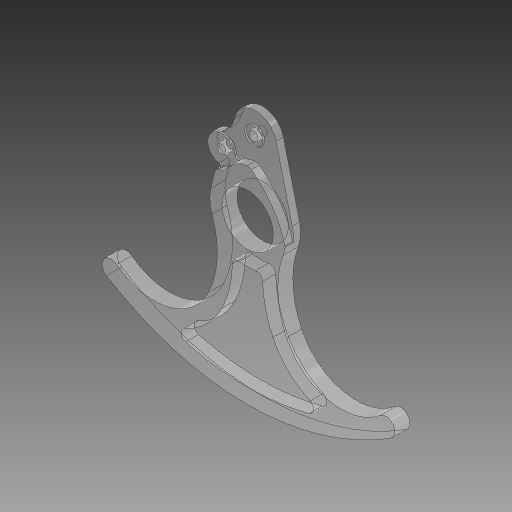
# Autodesk Inventor part: ヘッケン2
Saved by Autodesk Inventor 2020 (Build 240168000, 168)
## iProperties
Created: 2019-09-03
Part Number: ヘッケン2
Material: ポリカーボネート、クリア
Document SubType Name: Modeling
Designer: 雪村
Density: 1.2 g/cm^3
Appearance: ポリカーボネート - クリア
Mass: 9.36853 g
Surface Area: 71.3184 cm^2
Volume: 7.80711 cm^3
Description: ポリカ 5t
Author: 雪村
Autodesk Inventor part; units mm, degrees
ref_plane "YZ Plane" through (0, 0, 0) normal (1, 0, 0) x (0, 1, 0)
ref_plane "XZ Plane" through (0, 0, 0) normal (0, 1, 0) x (-1, 0, 0)
ref_plane "XY Plane" through (0, 0, 0) normal (0, 0, 1) x (1, 0, 0)
sketch "スケッチ1" plane through (0, 0, 0) normal (0, 0, 1) x (1, 0, 0)
  spline S0 degree 4 poles (47.3109, -61.9649) (47.0065, -62.1545) (46.5798, -62.4175) (46.0301, -62.7516) (45.3565, -63.1534) (44.8664, -63.4421) (44.3758, -63.7275) (43.8846, -64.0096) (43.3928, -64.2883) (42.9004, -64.5638) (42.4073, -64.8361) (41.9135, -65.1051) (41.419, -65.3708) (40.9238, -65.6334) (40.4279, -65.8927) (39.9312, -66.1487) (39.4337, -66.4016) (38.9355, -66.6513) (38.4364, -66.8977) (37.9366, -67.141) (37.4359, -67.381) (36.9344, -67.6179) (36.432, -67.8515) (35.9288, -68.082) (35.4247, -68.3093) (34.9198, -68.5333) (34.414, -68.7542) (33.9073, -68.9719) (33.3998, -69.1863) (32.8914, -69.3976) (32.3821, -69.6056) (31.8719, -69.8105) (31.3609, -70.0121) (30.849, -70.2105) (30.3362, -70.4056) (29.8225, -70.5976) (29.308, -70.7863) (28.7926, -70.9717) (28.2764, -71.1539) (27.7593, -71.3329) (27.2413, -71.5086) (26.7225, -71.681) (26.2029, -71.8502) (25.6825, -72.016) (25.1612, -72.1786) (24.6392, -72.3379) (24.1163, -72.4939) (23.5927, -72.6466) (23.0683, -72.796) (22.5431, -72.942) (22.0172, -73.0848) (21.4905, -73.2242) (20.9632, -73.3602) (20.4351, -73.4929) (19.9062, -73.6223) (19.3768, -73.7483) (18.8466, -73.8709) (18.3158, -73.9902) (17.7843, -74.1061) (17.2522, -74.2186) (16.7195, -74.3277) (16.1862, -74.4334) (15.6524, -74.5357) (15.1179, -74.6346) (14.5829, -74.73) (14.0474, -74.8221) (13.5114, -74.9107) (12.9749, -74.9959) (12.4379, -75.0777) (11.9005, -75.156) (11.3626, -75.2309) (10.8243, -75.3023) (10.2856, -75.3703) (9.7465, -75.4348) (9.207, -75.4958) (8.6672, -75.5534) (8.1271, -75.6075) (7.5867, -75.6581) (7.046, -75.7053) (6.505, -75.749) (5.9638, -75.7892) (5.4223, -75.8259) (4.8807, -75.8591) (4.3389, -75.8888) (3.7969, -75.915) (3.2547, -75.9378) (2.7124, -75.957) (2.1701, -75.9728) (1.6276, -75.985) (1.0851, -75.9937) (0.5426, -75.999) (0, -76.0007) (-0.5426, -75.999) (-1.0851, -75.9937) (-1.6276, -75.985) (-2.1701, -75.9728) (-2.7125, -75.957) (-3.2547, -75.9378) (-3.7969, -75.915) (-4.3389, -75.8888) (-4.8807, -75.8591) (-5.4224, -75.8259) (-5.9638, -75.7892) (-6.505, -75.749) (-7.046, -75.7053) (-7.5868, -75.6581) (-8.1272, -75.6075) (-8.6674, -75.5534) (-9.2072, -75.4958) (-9.7467, -75.4348) (-10.2859, -75.3703) (-10.8247, -75.3023) (-11.363, -75.2308) (-11.901, -75.156) (-12.4386, -75.0776) (-12.9757, -74.9959) (-13.5124, -74.9106) (-14.0486, -74.822) (-14.5843, -74.7299) (-15.1195, -74.6344) (-15.6541, -74.5355) (-16.1883, -74.4331) (-16.7219, -74.3274) (-17.2549, -74.2182) (-17.7874, -74.1057) (-18.3193, -73.9897) (-18.8505, -73.8704) (-19.3812, -73.7477) (-19.9113, -73.6216) (-20.4407, -73.4921) (-20.9695, -73.3593) (-21.4976, -73.2231) (-22.0251, -73.0835) (-22.5519, -72.9406) (-23.078, -72.7943) (-23.6035, -72.6447) (-24.1283, -72.4918) (-24.6524, -72.3355) (-25.1758, -72.1759) (-25.6985, -72.0129) (-26.2205, -71.8466) (-26.7418, -71.6771) (-27.2625, -71.5041) (-27.7825, -71.3279) (-28.3017, -71.1484) (-28.8203, -70.9655) (-29.3383, -70.7793) (-29.8555, -70.5898) (-30.3721, -70.397) (-30.8881, -70.2009) (-31.4034, -70.0014) (-31.9181, -69.7986) (-32.4322, -69.5925) (-32.9457, -69.3831) (-33.4587, -69.1703) (-33.9711, -68.9541) (-34.483, -68.7346) (-34.9944, -68.5118) (-35.5054, -68.2855) (-36.0159, -68.0558) (-36.526, -67.8228) (-37.0357, -67.5863) (-37.5452, -67.3463) (-38.0543, -67.1029) (-38.5633, -66.8559) (-39.072, -66.6054) (-39.5807, -66.3514) (-40.0892, -66.0938) (-40.5978, -65.8326) (-41.1064, -65.5676) (-41.6152, -65.299) (-42.1242, -65.0266) (-42.6335, -64.7504) (-43.1431, -64.4703) (-43.6533, -64.1863) (-44.164, -63.8983) (-44.6755, -63.6062) (-45.3809, -63.1982) (-45.9582, -62.8581) (-46.4075, -62.5897) (-46.7287, -62.3958) knots 0 0 0 0 0 0.014153 0.019804 0.025448 0.031087 0.03672 0.042347 0.047969 0.053586 0.059197 0.064804 0.070407 0.076005 0.081599 0.087189 0.092776 0.098358 0.103937 0.109513 0.115086 0.120655 0.126222 0.131786 0.137347 0.142906 0.148462 0.154016 0.159567 0.165117 0.170664 0.17621 0.181753 0.187295 0.192835 0.198374 0.203911 0.209447 0.214981 0.220514 0.226045 0.231576 0.237105 0.242633 0.24816 0.253686 0.259211 0.264735 0.270259 0.275781 0.281303 0.286824 0.292344 0.297864 0.303383 0.308902 0.31442 0.319937 0.325454 0.33097 0.336486 0.342002 0.347517 0.353031 0.358546 0.36406 0.369573 0.375087 0.3806 0.386112 0.391625 0.397137 0.402649 0.408161 0.413673 0.419184 0.424696 0.430207 0.435718 0.441229 0.446739 0.45225 0.457761 0.463271 0.468782 0.474292 0.479802 0.485312 0.490823 0.496333 0.501843 0.507353 0.512863 0.518373 0.523883 0.529394 0.534904 0.540414 0.545925 0.551435 0.556946 0.562456 0.567967 0.573478 0.578989 0.584501 0.590012 0.595524 0.601036 0.606548 0.61206 0.617573 0.623086 0.628599 0.634113 0.639627 0.645141 0.650656 0.656172 0.661687 0.667204 0.672721 0.678238 0.683757 0.689275 0.694795 0.700315 0.705837 0.711359 0.716882 0.722406 0.727931 0.733457 0.738984 0.744513 0.750043 0.755574 0.761107 0.766641 0.772178 0.777715 0.783255 0.788797 0.794341 0.799887 0.805435 0.810986 0.816539 0.822096 0.827655 0.833217 0.838783 0.844352 0.849924 0.855501 0.861082 0.866667 0.872256 0.877851 0.88345 0.889055 0.894666 0.900282 0.905905 0.911535 0.917171 0.922816 0.928468 0.934129 0.939798 0.945477 0.951166 0.956865 0.962575 0.968297 0.974032 0.979779 0.985541 1 1 1 1 1
  circle A0 centre (0, 0) radius 1.5
  circle A1 centre (0, -23) radius 8.525
  circle A2 centre (0, 0) radius 7.025
  circle A3 centre (0, -23) radius 12.525
  line L0 (-6.8212, 1.6799) -> (-12.1616, -20.0049)
  line L1 (6.8212, 1.6799) -> (12.1616, -20.0049)
  arc A4 (-43.3371, -57.4602) -> (-46.7287, -62.3958) centre (-45.1853, -59.8233) ccw
  arc A5 (47.3109, -61.9649) -> (43.8031, -57.1163) centre (45.732, -59.414) ccw
  line L2 (-46.7287, -62.3958) -> (-46.2133, -62.705) construction
  line L3 (46.8227, -62.2671) -> (47.3109, -61.9649) construction
  arc A6 (-43.3371, -57.4602) -> (-12.9977, -50.3865) centre (-31.0158, -41.7063) ccw
  arc A7 (-12.9977, -50.3865) -> (-11.7886, -27.2313) centre (-40.0249, -37.3662) ccw
  arc A8 (11.7739, -27.272) -> (12.8817, -50.3865) centre (39.975, -37.5042) ccw
  arc A9 (12.8817, -50.3865) -> (43.8031, -57.1163) centre (30.9439, -41.7983) ccw
  line L4 (-46.7287, -62.3958) -> (0, -23) construction
  line L5 (47.3109, -61.9649) -> (0, -23) construction
  line L6 (0, -23) -> (0, -76) construction
  point P0 (46.3342, -62.5658)
  point P1 (45.8451, -62.8612)
  point P2 (45.3556, -63.1532)
  point P3 (44.8656, -63.4419)
  point P4 (44.375, -63.7272)
  point P5 (43.8838, -64.0093)
  point P6 (43.392, -64.288)
  point P7 (42.8996, -64.5635)
  point P8 (42.4065, -64.8358)
  point P9 (41.9128, -65.1047)
  point P10 (41.4183, -65.3705)
  point P11 (40.9231, -65.633)
  point P12 (40.4272, -65.8923)
  point P13 (39.9305, -66.1483)
  point P14 (39.4331, -66.4012)
  point P15 (38.9348, -66.6508)
  point P16 (38.4358, -66.8973)
  point P17 (37.936, -67.1405)
  point P18 (37.4353, -67.3805)
  point P19 (36.9338, -67.6174)
  point P20 (36.4314, -67.851)
  point P21 (35.9282, -68.0815)
  point P22 (35.4242, -68.3087)
  point P23 (34.9193, -68.5328)
  point P24 (34.4135, -68.7537)
  point P25 (33.9068, -68.9713)
  point P26 (33.3993, -69.1858)
  point P27 (32.8909, -69.397)
  point P28 (32.3816, -69.6051)
  point P29 (31.8715, -69.8099)
  point P30 (31.3605, -70.0115)
  point P31 (30.8485, -70.2099)
  point P32 (30.3358, -70.4051)
  point P33 (29.8221, -70.597)
  point P34 (29.3076, -70.7857)
  point P35 (28.7922, -70.9711)
  point P36 (28.276, -71.1533)
  point P37 (27.7589, -71.3323)
  point P38 (27.241, -71.508)
  point P39 (26.7222, -71.6804)
  point P40 (26.2026, -71.8495)
  point P41 (25.6822, -72.0154)
  point P42 (25.1609, -72.178)
  point P43 (24.6389, -72.3373)
  point P44 (24.1161, -72.4933)
  point P45 (23.5924, -72.6459)
  point P46 (23.068, -72.7953)
  point P47 (22.5429, -72.9414)
  point P48 (22.0169, -73.0841)
  point P49 (21.4903, -73.2235)
  point P50 (20.9629, -73.3596)
  point P51 (20.4348, -73.4923)
  point P52 (19.906, -73.6216)
  point P53 (19.3765, -73.7476)
  point P54 (18.8464, -73.8702)
  point P55 (18.3156, -73.9895)
  point P56 (17.7841, -74.1054)
  point P57 (17.252, -74.2179)
  point P58 (16.7193, -74.327)
  point P59 (16.1861, -74.4327)
  point P60 (15.6522, -74.535)
  point P61 (15.1178, -74.6339)
  point P62 (14.5828, -74.7293)
  point P63 (14.0473, -74.8214)
  point P64 (13.5113, -74.91)
  point P65 (12.9748, -74.9952)
  point P66 (12.4378, -75.077)
  point P67 (11.9003, -75.1553)
  point P68 (11.3625, -75.2302)
  point P69 (10.8242, -75.3016)
  point P70 (10.2855, -75.3696)
  point P71 (9.7464, -75.4341)
  point P72 (9.2069, -75.4951)
  point P73 (8.6671, -75.5527)
  point P74 (8.127, -75.6068)
  point P75 (7.5866, -75.6574)
  point P76 (7.0459, -75.7046)
  point P77 (6.5049, -75.7482)
  point P78 (5.9637, -75.7884)
  point P79 (5.4223, -75.8251)
  point P80 (4.8806, -75.8583)
  point P81 (4.3388, -75.8881)
  point P82 (3.7968, -75.9143)
  point P83 (3.2547, -75.937)
  point P84 (2.7124, -75.9563)
  point P85 (2.1701, -75.972)
  point P86 (1.6276, -75.9843)
  point P87 (1.0851, -75.993)
  point P88 (0.5426, -75.9983)
  point P89 (-0.5426, -75.9983)
  point P90 (-1.0851, -75.993)
  point P91 (-1.6276, -75.9843)
  point P92 (-2.1701, -75.972)
  point P93 (-2.7124, -75.9563)
  point P94 (-3.2547, -75.937)
  point P95 (-3.7968, -75.9143)
  point P96 (-4.3388, -75.8881)
  point P97 (-4.8806, -75.8583)
  point P98 (-5.4223, -75.8251)
  point P99 (-5.9637, -75.7884)
  point P100 (-6.505, -75.7482)
  point P101 (-7.046, -75.7046)
  point P102 (-7.5867, -75.6574)
  point P103 (-8.1271, -75.6068)
  point P104 (-8.6673, -75.5527)
  point P105 (-9.2071, -75.4951)
  point P106 (-9.7466, -75.434)
  point P107 (-10.2858, -75.3695)
  point P108 (-10.8245, -75.3016)
  point P109 (-11.3629, -75.2301)
  point P110 (-11.9009, -75.1553)
  point P111 (-12.4384, -75.0769)
  point P112 (-12.9755, -74.9951)
  point P113 (-13.5122, -74.9099)
  point P114 (-14.0484, -74.8213)
  point P115 (-14.5841, -74.7292)
  point P116 (-15.1193, -74.6337)
  point P117 (-15.6539, -74.5348)
  point P118 (-16.1881, -74.4324)
  point P119 (-16.7217, -74.3267)
  point P120 (-17.2547, -74.2175)
  point P121 (-17.7872, -74.105)
  point P122 (-18.319, -73.9891)
  point P123 (-18.8503, -73.8697)
  point P124 (-19.381, -73.747)
  point P125 (-19.911, -73.6209)
  point P126 (-20.4404, -73.4914)
  point P127 (-20.9692, -73.3586)
  point P128 (-21.4973, -73.2224)
  point P129 (-22.0248, -73.0828)
  point P130 (-22.5516, -72.9399)
  point P131 (-23.0777, -72.7937)
  point P132 (-23.6031, -72.6441)
  point P133 (-24.1279, -72.4911)
  point P134 (-24.652, -72.3348)
  point P135 (-25.1754, -72.1752)
  point P136 (-25.6981, -72.0123)
  point P137 (-26.2201, -71.846)
  point P138 (-26.7414, -71.6764)
  point P139 (-27.2621, -71.5035)
  point P140 (-27.782, -71.3273)
  point P141 (-28.3013, -71.1478)
  point P142 (-28.8199, -70.9649)
  point P143 (-29.3378, -70.7788)
  point P144 (-29.855, -70.5893)
  point P145 (-30.3716, -70.3965)
  point P146 (-30.8875, -70.2003)
  point P147 (-31.4028, -70.0009)
  point P148 (-31.9175, -69.7981)
  point P149 (-32.4316, -69.592)
  point P150 (-32.9451, -69.3826)
  point P151 (-33.458, -69.1698)
  point P152 (-33.9704, -68.9537)
  point P153 (-34.4823, -68.7342)
  point P154 (-34.9937, -68.5113)
  point P155 (-35.5046, -68.2851)
  point P156 (-36.0151, -68.0554)
  point P157 (-36.5252, -67.8224)
  point P158 (-37.0349, -67.5859)
  point P159 (-37.5443, -67.346)
  point P160 (-38.0534, -67.1025)
  point P161 (-38.5623, -66.8556)
  point P162 (-39.071, -66.6052)
  point P163 (-39.5796, -66.3512)
  point P164 (-40.0881, -66.0936)
  point P165 (-40.5967, -65.8324)
  point P166 (-41.1053, -65.5675)
  point P167 (-41.614, -65.2989)
  point P168 (-42.1229, -65.0265)
  point P169 (-42.6321, -64.7504)
  point P170 (-43.1417, -64.4703)
  point P171 (-43.6518, -64.1864)
  point P172 (-44.1625, -63.8984)
  point P173 (-44.6739, -63.6064)
  point P174 (-45.186, -63.3102)
  point P175 (-45.6991, -63.0098)
  dimension "d0" = 3
  dimension "d1" = 14.05
  dimension "d2" = 23
  dimension "d3" = 17.05
  dimension "d4" = 4
  dimension "d5" = 3
  dimension "d6" = 3
  dimension "d7" = 20
  dimension "d9" = 20
  dimension "d10" = 30
  dimension "d11" = 30
  dimension "d12" = 20
  dimension "d64" = 61.291
  dimension "d65" = 61.1195
  constraints: 18 point on circle, 14 end point, 12 tangent, 10 centre point, 3 coincident, 1 horizontal alignment, 1 point on line, 1 vertical alignment, 364 other
  measures "d0" diameter of A0
  measures "d1" diameter of A2
  measures "d2" distance of A1.centre point (0, 0)
  measures "d3" diameter of A1
  measures "d4" radial gap between concentric circles of A1 A3
  measures "d5" radius of A4
  measures "d6" radius of A5
  measures "d7" radius of A6
  measures "d9" radius of A9
  measures "d10" radius of A8
  measures "d11" radius of A7
  measures "d64" distance of L3.end L4.end
  measures "d65" distance of L2.start L4.end
extrude "押し出し1" add sketch "スケッチ1" along normal blind 5
sketch "スケッチ2" plane through (0, 0, 5) normal (0, 0, 1) x (1, 0, 0)
  line L0 (0, 0) -> (-10.6688, -9.0652)
  circle A0 centre (-10.6688, -9.0652) radius 1.5
  circle A1 centre (0, 0) radius 1.5
  circle A2 centre (-10.6688, -9.0652) radius 4.025
  circle A3 centre (0, 0) radius 7.025
  arc A4 (0.3692, -7.0153) -> (-7.3502, -11.3428) centre (0.8948, -17.0015) ccw
  arc A5 (-12.3807, -5.4224) -> (-6.8636, 1.497) centre (-16.6339, 3.628) ccw
  circle A6 centre (0, -23) radius 8.525
  arc A7 (0.3955, -7.5146) -> (-6.9379, -11.6257) centre (0.8948, -17.0015) ccw
  circle A8 centre (0, 0) radius 7.525
  circle A9 centre (-10.6688, -9.0652) radius 4.525
  circle A10 centre (0, -23) radius 8.525 projected
  circle A11 centre (0, 0) radius 1.5 projected
  circle A12 centre (0, 0) radius 3
  arc A13 (6.8212, 1.6799) -> (-6.8212, 1.6799) centre (0, 0) ccw projected
  point P0 (-6.2404, -9.995)
  point P1 (-6.9379, -11.6257)
  point P2 (0.3955, -7.5146)
  point P3 (-7.5105, -0.4663)
  point P4 (-10.8715, -4.5447)
  point P5 (-5.7345, -4.8725)
  point P6 (-7.5105, -0.4663)
  point P7 (-7.6015, -6.4589)
  point P8 (-5.3534, -4.5488)
  point P9 (-10.8715, -4.5447)
  point P10 (-6.2404, -9.995)
  dimension "d15" = 14
  dimension "d16" = 3
  dimension "d17" = 8.05
  dimension "d18" = 14.05
  dimension "d19" = 10
  dimension "d20" = 10
  dimension "d21" = 5
  dimension "d23" = 0.5
  dimension "d24" = 0.5
  dimension "d25" = 0.5
  dimension "d26" = 6
  constraints: 10 point on circle, 9 centre point, 6 tangent, 5 coincident, 2 concentric, 2 end point, 6 other
  measures "d15" distance of L0.start L0.end
  measures "d16" diameter of A0
  measures "d17" diameter of A2
  measures "d18" diameter of A3
  measures "d19" radius of A5
  measures "d20" radius of A4
  measures "d23" radial gap between concentric circles of A4 A7
  measures "d26" diameter of A12
extrude "押し出し2" cut sketch "スケッチ2" against normal through all contours A0
extrude "押し出し3" add sketch "スケッチ2" against normal blind 5 contours L0 A8 A5 A3 | L0 A9 A5 A8 | L0 A2 A5 A9 | A2 | A5 A2 A4 A9
extrude "押し出し4" cut sketch "スケッチ2" against normal blind 2.6 contours A3 A4 A8 L0 | L0 A8 A5 A3 | A3 | A8 A4 A9 L0 | L0 A9 A5 A8
extrude "押し出し5" cut sketch "スケッチ2" against normal blind 2.6 contours A5 A8 A4 A3 | A8 A7 A9 A4
extrude "押し出し6" cut sketch "スケッチ2" against normal blind 2 contours A9 A4 A2 L0 | L0 A2 A5 A9 | A2 | A5 A2 A4 A9 | A0 | A12
sketch "スケッチ3" plane through (0, 0, 5) normal (0, 0, 1) x (1, 0, 0)
  circle A0 centre (0, 0) radius 1.5
  circle A1 centre (0, -23) radius 8.525
  arc A2 (13.5102, -34.0119) -> (26.3695, -30.4286) centre (20.528, -34.3308) ccw
  line L0 (26.3695, -30.4286) -> (7.5291, -2.2246)
  arc A3 (9.0465, 2.5403) -> (7.5291, -2.2246) centre (10.1892, -0.4476) ccw
  arc A4 (9.0465, 2.5403) -> (7.7583, 7.344) centre (8.1536, 4.8754) ccw
  line L1 (7.7583, 7.344) -> (-0.9526, 5.9492)
  arc A5 (-0.9526, 5.9492) -> (-2.8348, -5.3165) centre (0, 0) ccw
  arc A6 (13.5102, -34.0119) -> (-2.8348, -5.3165) centre (-17.3869, -32.6082) ccw
  circle A7 centre (0, 0) radius 4.025
  circle A8 centre (20.528, -34.3308) radius 4.025
  line L2 (8.1536, 4.8754) -> (0, 0)
  line L3 (0, 0) -> (20.528, -34.3308)
  line L4 (0, 0) -> (0, -23)
  line L5 (0, -23) -> (-14.8833, -14.7849)
  line L6 (-14.8833, -14.7849) -> (20.528, -34.3308)
  arc A9 (-1.0316, 6.4429) -> (-3.07, -5.7577) centre (0, 0) ccw
  line L7 (-1.0316, 6.4429) -> (7.6793, 7.8377)
  arc A10 (9.2251, 2.0733) -> (7.6793, 7.8377) centre (8.1536, 4.8754) ccw
  arc A11 (9.2251, 2.0733) -> (7.9449, -1.9469) centre (10.1892, -0.4476) ccw
  line L8 (7.9449, -1.9469) -> (26.7853, -30.1508)
  arc A12 (13.0108, -33.9892) -> (26.7853, -30.1508) centre (20.528, -34.3308) ccw
  arc A13 (13.0108, -33.9892) -> (-3.07, -5.7577) centre (-17.3869, -32.6082) ccw
  arc A14 (0.3955, -7.5146) -> (-6.9379, -11.6257) centre (0.8948, -17.0015) ccw projected
  arc A15 (0.3955, -7.5146) -> (7.4662, -0.9391) centre (0, 0) ccw projected
  point P0 (0, -7.6358)
  point P1 (12.9421, -30.1436)
  point P2 (13.4655, -30.4325)
  point P3 (0, -7.0289)
  point P4 (0, -7.6358)
  point P5 (0, -7.0289)
  point P6 (13.4655, -30.4325)
  point P7 (12.9421, -30.1436)
  point P8 (-0.1161, -7.5554)
  point P9 (0.6672, -7.4954)
  dimension "d37" = 8.05
  dimension "d38" = 30.929
  dimension "d39" = 8.05
  dimension "d40" = 3
  dimension "d41" = 2.5
  dimension "d42" = 3.199
  dimension "d43" = 40
  dimension "d44" = 9.5
  dimension "d45" = 90
  dimension "d46" = 33.9179
  dimension "d47" = 17
  dimension "d48" = 40.4475
  dimension "d49" = 0.5
  dimension "d50" = 2
  constraints: 20 point on circle, 18 end point, 14 centre point, 7 tangent, 2 concentric, 1 coincident, 1 collinear, 1 vertical, 8 other
  measures "d37" diameter of A7
  measures "d38" radius of A6
  measures "d39" diameter of A8
  measures "d40" radial gap between concentric circles of A2 A8
  measures "d41" radius of A4
  measures "d42" radius of A3
  measures "d43" distance of A2.centre L2.end
  measures "d44" distance of A5.centre L2.start
  measures "d45" angle of L3 L2
  measures "d46" distance of L0.start L0.end
  measures "d47" distance of L4.end L5.end
  measures "d48" distance of L5.end L3.end
  measures "d49" radial gap between concentric circles of A6 A13
  measures "d50" radial gap between concentric circles of A5 A7
extrude "押し出し7" cut sketch "スケッチ3" against normal blind 2.6 contours A7 L4 A6 A5 L1 A4 A3 A15 L3 | L3 A15 A6 L4 A7 | A15 A3 L0 A2 A6 L6 A8 L3 | L3 A8 L6 A6 A15 | L4 A14 A13 A9 L7 A10 A11 L8 A12 L6 A6 A2 L0 A3 A4 L1 A5 | A6 A15 A14 L4
sketch "スケッチ4" plane through (0, 0, 5) normal (0, 0, 1) x (1, 0, 0)
  arc A0 (-43.3371, -57.4602) -> (-12.9977, -50.3865) centre (-31.0158, -41.7063) ccw projected
  arc A1 (-43.3371, -57.4602) -> (-46.7287, -62.3958) centre (-45.1853, -59.8233) ccw projected
  spline S0 degree 5 poles (-46.7287, -62.3958) (-42.286, -65.0772) (-37.8291, -67.4223) (-33.2662, -69.4678) (-28.606, -71.1867) (-19.1173, -73.9516) (-14.2885, -74.9975) (-9.3966, -75.6914) (-4.4706, -76.0253) (5.3761, -75.9723) (10.2982, -75.5854) (15.183, -74.8391) (20.0004, -73.7422) (29.452, -70.8796) (34.0867, -69.1138) (38.6089, -67.0279) (43.0091, -64.6436) (47.3109, -61.9649) knots 0 0 0 0 0 0 0.25 0.25 0.25 0.25 0.5 0.5 0.5 0.5 0.75 0.75 0.75 0.75 1 1 1 1 1 1
  arc A2 (-12.9977, -50.3865) -> (-11.7886, -27.2313) centre (-40.0249, -37.3662) ccw projected
  arc A3 (11.7739, -27.272) -> (12.8817, -50.3865) centre (39.975, -37.5042) ccw projected
  arc A4 (12.8817, -50.3865) -> (43.8031, -57.1163) centre (30.9439, -41.7983) ccw projected
  arc A5 (47.3109, -61.9649) -> (43.8031, -57.1163) centre (45.732, -59.414) ccw projected
  circle A6 centre (0, -23) radius 8.525 projected
  circle A7 centre (0, -23) radius 13.525
  arc A8 (-8.4931, -52.5566) -> (-7.0826, -25.5422) centre (-40.0249, -37.3662) ccw
  arc A9 (-26.8528, -66.3572) -> (-8.4931, -52.5566) centre (-31.0158, -41.7063) ccw
  arc A10 (8.3662, -52.5336) -> (26.6466, -66.4262) centre (30.9439, -41.7983) ccw
  arc A11 (7.0738, -25.5666) -> (8.3662, -52.5336) centre (39.975, -37.5042) ccw
  spline S1 degree 5 poles (-26.8528, -66.3572) (-21.6067, -68.2038) (-16.21, -69.6222) (-10.6996, -70.57) (0.2143, -71.4698) (11.1188, -70.4896) (16.411, -69.5575) (21.5987, -68.1919) (26.6466, -66.4262) knots 0 0 0 0 0 0 0.509801 0.509801 0.509801 1 1 1 1 1 1
  point P0 (0, 0)
  point P1 (5.0293, -35.5551)
  point P2 (-5.0727, -35.5377)
  dimension "d53" = 5
  dimension "d54" = 5
  constraints: 8 point on circle, 5 centre point, 2 concentric, 6 other
  measures "d53" radial gap between concentric circles of A6 A7
  measures "d54" radial gap between concentric circles of A2 A8
extrude "押し出し8" cut sketch "スケッチ4" against normal through all contours A7 A11 A10 S1 A9 A8
fillet "フィレット1" radius 2 5 edges at (0.6672, -7.4954, 3.7) (-26.8528, -66.3572, 2.5) (26.6466, -66.4262, 2.5) (-5.0727, -35.5377, 2.5) (5.0293, -35.5551, 2.5)
fillet "フィレット1" radius 1 4 edges at (-10.8715, -4.5447, 1.2) (-10.5816, -13.5893, 1.5) (-10.5816, -13.5893, 4) (12.4426, -24.4346, 3.7)
sketch "スケッチ6" plane through (0, 0, 0) normal (0, 0, -1) x (-1, 0, 0)
  spline S0 degree 6 poles (20.543, -68.3033) (20.4471, -68.3288) (20.3511, -68.3541) (20.2552, -68.3793) (20.1592, -68.4043) (20.0631, -68.4292) (16.6745, -69.3023) (13.3396, -69.9869) (9.972, -70.5017) (6.5823, -70.8431) (3.1816, -71.009) (-2.464, -70.9935) (-4.7093, -70.9108) (-6.9511, -70.7517) (-9.1863, -70.5165) (-11.4115, -70.2059) (-14.7569, -69.6241) (-15.8865, -69.4075) (-17.0124, -69.1717) (-18.1341, -68.9166) (-19.2512, -68.6427) (-20.3633, -68.35) knots 0 0 0 0 0 0 0 0.014391 0.014391 0.014391 0.014391 0.014391 0.50752 0.50752 0.50752 0.50752 0.50752 0.833202 0.833202 0.833202 0.833202 0.833202 1 1 1 1 1 1 1 projected
  spline S1 degree 2 poles (-20.6758, -64.5923) (-25.8259, -66.9123) (-20.3633, -68.35) knots 0 0 0 1 1 1 weights 1 0.333769 1 projected
  arc A0 (-20.6758, -64.5923) -> (-8.3662, -52.5336) centre (-30.9439, -41.7983) ccw projected
  arc A1 (-8.3662, -52.5336) -> (-4.9819, -38.1963) centre (-39.975, -37.5042) ccw projected
  arc A2 (-2.5981, -36.2731) -> (-4.9819, -38.1963) centre (-2.9823, -38.2359) ccw projected
  arc A3 (-2.5981, -36.2731) -> (2.6439, -36.2641) centre (0, -23) ccw projected
  arc A4 (5.0343, -38.179) -> (2.6439, -36.2641) centre (3.0348, -38.2255) ccw projected
  arc A5 (5.0343, -38.179) -> (8.4931, -52.5566) centre (40.0249, -37.3662) ccw projected
  arc A6 (8.4931, -52.5566) -> (20.8436, -64.5432) centre (31.0158, -41.7063) ccw projected
  spline S2 degree 2 poles (20.543, -68.3033) (26.0211, -66.8494) (20.8437, -64.5433) knots 0 0 0 1 1 1 weights 1 0.332762 1 projected
  line L0 (6.8212, 1.6799) -> (7.0133, 0.8997) projected
  arc A7 (6.8212, 1.6799) -> (-6.8212, 1.6799) centre (0, 0) ccw projected
  line L1 (-12.1616, -20.0049) -> (-6.8212, 1.6799) projected
  arc A8 (-12.1616, -20.0049) -> (-11.7739, -27.272) centre (0, -23) ccw projected
  arc A9 (-12.8817, -50.3865) -> (-11.7739, -27.272) centre (-39.975, -37.5042) ccw projected
  arc A10 (-43.8031, -57.1163) -> (-12.8817, -50.3865) centre (-30.9439, -41.7983) ccw projected
  arc A11 (-43.8031, -57.1163) -> (-47.3109, -61.9649) centre (-45.732, -59.414) ccw projected
  arc A12 (46.7287, -62.3958) -> (43.3371, -57.4602) centre (45.1853, -59.8233) ccw projected
  arc A13 (12.9977, -50.3865) -> (43.3371, -57.4602) centre (31.0158, -41.7063) ccw projected
  arc A14 (11.7886, -27.2313) -> (12.9977, -50.3865) centre (40.0249, -37.3662) ccw projected
  arc A15 (11.7886, -27.2313) -> (12.1616, -20.0049) centre (0, -23) ccw projected
  line L2 (10.8567, -14.7064) -> (12.1616, -20.0049) projected
  arc A16 (11.6179, -13.4895) -> (10.8567, -14.7064) centre (11.8277, -14.4672) ccw projected
  arc A17 (11.6179, -13.4895) -> (11.1281, -4.5635) centre (10.6688, -9.0652) ccw projected
  arc A18 (10.6291, -4.3683) -> (11.1281, -4.5635) centre (11.2296, -3.5687) ccw projected
  arc A19 (7.0133, 0.8997) -> (10.6291, -4.3683) centre (16.6339, 3.628) ccw projected
  circle A20 centre (10.6688, -9.0652) radius 1.5 projected
  circle A21 centre (0, 0) radius 1.5 projected
  circle A22 centre (0, -23) radius 8.525 projected
  constraints: 4 other
extrude "押し出し10" add sketch "スケッチ6" against normal blind 0.7 contours S0 S1 A0 A1 A2 A3 A4 A5 A6 S2
fillet "フィレット2" radius 1 1 edges at (-6.9379, -11.6257, 2.7)
sketch "スケッチ9" plane through (0, 0, 5) normal (0, 0, 1) x (1, 0, 0)
  circle A0 centre (0, 0) radius 3 projected
  arc A1 (12.417, -24.6409) -> (14.4989, -24.916) centre (13.458, -24.7785) ccw
  arc A2 (-11.8705, -2.6743) -> (-9.0431, 1.4395) centre (-16.6339, 3.628) ccw
  line L0 (-9.0431, 1.4395) -> (-8.8603, 2.1821)
  arc A3 (8.8603, 2.1821) -> (-8.8603, 2.1821) centre (0, 0) ccw
  line L1 (8.8603, 2.1821) -> (14.2007, -19.5027)
  arc A4 (14.4989, -24.916) -> (14.2007, -19.5027) centre (0, -23) ccw
  arc A5 (12.417, -24.6409) -> (12.3884, -24.2393) centre (11.4257, -24.5099) ccw projected
  arc A6 (12.3884, -24.2393) -> (1.2855, -7.9517) centre (-17.3869, -32.6082) ccw projected
  arc A7 (1.2855, -7.9517) -> (-0.1397, -7.558) centre (0.0781, -9.5461) ccw projected
  arc A8 (-0.1397, -7.558) -> (-4.6011, -9.2526) centre (0.8948, -17.0015) ccw projected
  arc A9 (-6.1731, -8.5506) -> (-4.6011, -9.2526) centre (-5.1796, -8.4369) ccw projected
  arc A10 (-6.1731, -8.5506) -> (-11.1281, -4.5635) centre (-10.6688, -9.0652) ccw projected
  arc A11 (-11.8705, -2.6743) -> (-11.1281, -4.5635) centre (-11.2351, -3.5151) ccw
  constraints: 12 point on circle, 6 centre point, 4 end point, 3 tangent, 6 other
